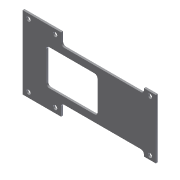
# Autodesk Inventor part: bottom support extension
Saved by Autodesk Inventor 2011 (Build 150239000, 239)
## iProperties
Created: 2011-06-09
Part Number: bottom support extension
Document SubType Name: Modeling
Designer: ijs09
Density: 1 g/cm^3
Author: ijs09
Autodesk Inventor part; units mm, degrees
ref_plane "YZ Plane" through (0, 0, 0) normal (1, 0, 0) x (0, 1, 0)
ref_plane "XZ Plane" through (0, 0, 0) normal (0, 1, 0) x (-1, 0, 0)
ref_plane "XY Plane" through (0, 0, 0) normal (0, 0, 1) x (1, 0, 0)
sketch "Sketch1" plane through (0, 0, 0) normal (0, 0, 1) x (1, 0, 0)
  circle A0 centre (91.8298, -26) radius 2.15
  circle A1 centre (91.8298, 26) radius 2.15
  line L0 (1.8298, 37) -> (-37.1702, 37)
  line L1 (-37.1702, 37) -> (-37.1702, -37)
  line L2 (-37.1702, -37) -> (1.8298, -37)
  circle A2 centre (-4.1702, -32) radius 2.15
  circle A3 centre (-31.1702, -32) radius 2.15
  circle A4 centre (-31.1702, 32) radius 2.15
  circle A5 centre (-4.1702, 32) radius 2.15
  line L3 (-9.9952, 18) -> (35.6548, 18)
  line L4 (38.8298, 14.825) -> (38.8298, -14.825)
  line L5 (35.6548, -18) -> (-9.9952, -18)
  line L6 (-13.1702, -14.825) -> (-13.1702, 14.825)
  arc A6 (-9.9952, 18) -> (-13.1702, 14.825) centre (-9.9952, 14.825) ccw
  arc A7 (-13.1702, -14.825) -> (-9.9952, -18) centre (-9.9952, -14.825) ccw
  arc A8 (38.8298, 14.825) -> (35.6548, 18) centre (35.6548, 14.825) ccw
  arc A9 (35.6548, -18) -> (38.8298, -14.825) centre (35.6548, -14.825) ccw
  line L7 (85.8298, 28.175) -> (85.8298, 30)
  line L8 (85.8298, 30) -> (97.8298, 30)
  line L9 (97.8298, 30) -> (97.8298, -30)
  line L10 (85.8298, -28.175) -> (85.8298, -30)
  line L11 (85.8298, -30) -> (97.8298, -30)
  arc A10 (82.6548, 25) -> (85.8298, 28.175) centre (82.6548, 28.175) ccw
  arc A11 (85.8298, -28.175) -> (82.6548, -25) centre (82.6548, -28.175) ccw
  line L12 (1.8298, 37) -> (1.8298, 28.175)
  line L13 (5.0048, 25) -> (82.6548, 25)
  line L14 (1.8298, -37) -> (1.8298, -28.175)
  line L15 (5.0048, -25) -> (82.6548, -25)
  arc A12 (1.8298, 28.175) -> (5.0048, 25) centre (5.0048, 28.175) ccw
  arc A13 (5.0048, -25) -> (1.8298, -28.175) centre (5.0048, -28.175) ccw
  point P0 (0, 0)
  point P1 (85.8298, 26.8)
  dimension "d2" = 4.3
  dimension "d3" = 4.3
  dimension "d20" = 6
  dimension "d21" = 6
  dimension "d23" = 4.3
  dimension "d24" = 4.3
  dimension "d25" = 4.3
  dimension "d26" = 4.3
  dimension "d41" = 3.175
  dimension "d53" = 6
  dimension "d54" = 6
  dimension "d55" = 6
  dimension "d57" = 3.175
  dimension "d63" = 84
  dimension "d64" = 3.175
  dimension "d65" = 3.175
  dimension "d68" = 84
  dimension "d69" = 36
  dimension "d70" = 52
  dimension "d75" = 6
  dimension "d76" = 6
  dimension "d78" = 12
  dimension "d79" = 39
  dimension "d80" = 24
  dimension "d81" = 7
  dimension "d82" = 7
  dimension "d83" = 74
  dimension "d84" = 12
  dimension "d85" = 5
  dimension "d86" = 5
  dimension "d87" = 5
  dimension "d88" = 5
  dimension "d89" = 37
  dimension "d90" = 52
  dimension "d92" = 26
  dimension "d93" = 25
  dimension "d94" = 25
  dimension "d95" = 4
  dimension "d96" = 4
  constraints: 32 end point, 16 point on circle, 16 tangent, 14 centre point, 9 perpendicular, 6 coincident, 5 parallel, 4 equal radius, 1 horizontal, 1 point on line
  measures "d2" diameter of A1
  measures "d3" diameter of A0
  measures "d20" distance from line of point (-31.17, 32) L1
  measures "d21" distance from line of L1 point (-31.17, -32)
  measures "d23" diameter of A5
  measures "d24" diameter of A4
  measures "d25" diameter of A3
  measures "d26" diameter of A2
  measures "d41" radius of A6
  measures "d53" distance from line of L9 A1.centre
  measures "d54" distance from line of L7 point (91.83, 26)
  measures "d55" distance from line of L10 A0.centre
  measures "d57" radius of A10
  measures "d63" distance from line of L12 L7.end
  measures "d64" radius of A12
  measures "d65" radius of A13
  measures "d68" distance between parallel lines of L14 L10
  measures "d69" distance between parallel lines of L5 L3
  measures "d70" distance between parallel lines of L4 L6
  measures "d75" distance from line of L12 A5.centre
  measures "d76" distance from line of A2.centre L14
  measures "d78" distance from line of L9 L10.end
  measures "d79" distance between parallel lines of L1 L12
  measures "d80" distance between parallel lines of L1 L6
  measures "d81" distance between parallel lines of L3 L13
  measures "d82" distance between parallel lines of L15 L5
  measures "d83" distance between parallel lines of L2 L0
  measures "d84" distance between parallel lines of L13 L0
  measures "d85" distance from line of L0 A4.centre
  measures "d86" distance from line of L0 A5.centre
  measures "d87" distance from line of L2 point (-31.17, -32)
  measures "d88" distance from line of point (-4.17, -32) L2
  measures "d89" distance from line of point (0, 0) L2
  measures "d90" distance of A0.centre A1.centre
  measures "d92" vertical distance of point (0, 0) A0.centre
  measures "d93" distance from line of L15 point (0, 0)
  measures "d94" distance from line of L13 point (0, 0)
  measures "d95" distance from line of A1.centre L8
  measures "d96" distance from line of L11 A0.centre
extrude "Extrusion5" add sketch "Sketch1" along normal blind 2
equation "\"d3\" = d2"
equation "\"d20\" = d19"
equation "\"d21\" = d19"
equation "\"d24\" = d23"
equation "\"d25\" = d23"
equation "\"d26\" = d23"
equation "\"d54\" = d53"
equation "\"d55\" = d53"
equation "\"d68\" = d63"
equation "\"d75\" = d19"
equation "\"d76\" = d19"
equation "\"d19\" = 6"
body "Solid5"
